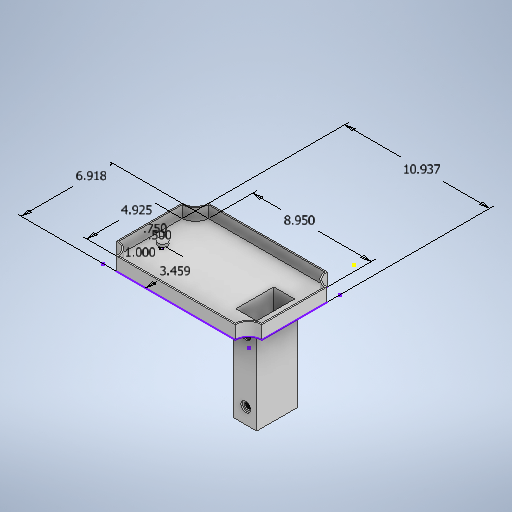
# Autodesk Inventor part: BASE
Saved by Autodesk Inventor 2025 (Build 290162010, 162A)
## iProperties
Created: 2024-07-31
Part Number: BASE
Material: Generic
Document SubType Name: Modeling
Designer: darkb
Density: 1 g/cm^3
Appearance: Default
Author: darkb
Autodesk Inventor part; units mm, degrees
ref_plane "YZ Plane" through (0, 0, 0) normal (1, 0, 0) x (0, 1, 0)
ref_plane "XZ Plane" through (0, 0, 0) normal (0, 1, 0) x (-1, 0, 0)
ref_plane "XY Plane" through (0, 0, 0) normal (0, 0, 1) x (1, 0, 0)
sketch "Sketch1" plane through (0, 0, 0) normal (0, 1, 0) x (-1, 0, 0)
  line L0 (217.0075, 238.5115) -> (-11.2469, 238.5115)
  line L1 (-36.6469, 213.1115) -> (-36.6469, 88.1828)
  line L2 (-11.5925, 62.7851) -> (215.7472, 62.7851)
  line L3 (241.1469, 88.0591) -> (241.1469, 213.1428)
  arc A0 (217.0075, 238.5115) -> (241.1469, 213.1428) centre (242.4075, 238.5115) ccw
  arc A1 (241.1469, 88.0591) -> (215.7472, 62.7851) centre (241.1469, 62.6591) ccw
  arc A2 (-36.6469, 213.1115) -> (-11.2469, 238.5115) centre (-36.6469, 238.5115) ccw
  arc A3 (-11.5925, 62.7851) -> (-36.6469, 88.1828) centre (-36.9925, 62.7851) ccw
  circle A4 centre (215.7469, 150.6529) radius 9.525
  circle A5 centre (215.7469, 150.6529) radius 6.35
  point P0 (0, 0)
  dimension "d6" = 227.3398
  dimension "d7" = 277.7939
  dimension "d10" = 125.0838
  dimension "d11" = 175.7264
  dimension "d12" = 19.05
  dimension "d13" = 12.7
  dimension "d14" = 87.8586
  dimension "d15" = 25.4
  constraints: 8 end point, 8 point on circle, 6 centre point, 2 parallel, 1 coincident, 1 horizontal, 1 perpendicular
  measures "d6" distance of L2.start L2.end
  measures "d7" distance between parallel lines of L1 L3
  measures "d10" distance of L3.start L3.end
  measures "d11" distance between parallel lines of L2 L0
  measures "d12" diameter of A4
  measures "d13" diameter of A5
  measures "d14" distance from line of L0 A4.centre
  measures "d15" distance from line of A4.centre L3
extrude "Extrusion1" add sketch "Sketch1" along normal blind 25.4 contours A0 L3 A1 L2 A3 L1 A2 L0 | A4 | A5
extrude "Extrusion2" cut sketch "Sketch1" along normal blind 5.08 contours A5
sketch "Sketch2" plane through (0, 0, 0) normal (0, -1, 0) x (1, 0, 0)
  point P0 (0, 0)
sketch "Sketch3" plane through (0, 0, 0) normal (0, -1, 0) x (1, 0, 0)
  line L0 (-39.8772, 113.6871) -> (5.2014, 113.6871)
  line L1 (5.2014, 113.6871) -> (5.2014, 191.46)
  line L2 (5.2014, 191.46) -> (-39.8772, 191.46)
  line L3 (-39.8772, 191.46) -> (-39.8772, 113.6871)
  point P0 (0, 0)
  constraints: 8 end point, 2 parallel, 1 horizontal, 1 perpendicular
extrude "Extrusion3" add sketch "Sketch3" along normal blind 177.8
sketch "Sketch4" plane through (-39.8772, 0, 191.46) normal (0, 0, 1) x (1, 0, 0)
  point P0 (39.8772, 0)
sketch "Sketch5" plane through (-39.8772, 0, 191.46) normal (0, 0, 1) x (1, 0, 0)
  circle A0 centre (24.2438, -148.3134) radius 6.35
  point P0 (39.8772, 0)
  dimension "d20" = 12.7
  constraints: 1 centre point
  measures "d20" diameter of A0
hole "Hole1" at (-15.6334, -148.3134, 191.46) direction (0, 0, -1) diameter 12.7 end through all counterbore diameter 19.05 counterbore depth 3.048
shell "Shell1" thickness 2.54 removed faces 2 at (-24.851, -177.8, 139.6114) at (-15.1224, -154.6429, 163.5037)
sketch "Sketch6" plane through (-39.8772, 0, 191.46) normal (0, 0, 1) x (1, 0, 0)
  circle A0 centre (24.2438, -27.5812) radius 6.35
  point P0 (39.8772, 0)
  dimension "d29" = 12.7
  constraints: 1 centre point
  measures "d29" diameter of A0
hole "Hole2" at (-15.6334, -27.5812, 191.46) direction (0, 0, -1) diameter 12.7 end through all counterbore diameter 19.05 counterbore depth 3.048
shell "Shell2" thickness 2.54 removed faces 3 at (-143.2625, 25.4, 176.3813) at (-140.9901, 22.86, 175.1392) at (-153.6846, 2.54, 191.1872)
body "Solid1"
